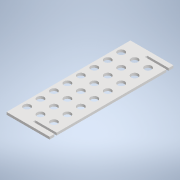
# Autodesk Inventor part: ChromoHolder
Saved by Autodesk Inventor 2020 (Build 240168000, 168)
## iProperties
Created: 2019-07-01
Part Number: ChromoHolder
Material: Generic
Document SubType Name: Modeling
Designer: eugen
Density: 1 g/cm^3
Appearance: Default
Author: eugen
Autodesk Inventor part; units mm, degrees
ref_plane "YZ Plane" through (0, 0, 0) normal (1, 0, 0) x (0, 1, 0)
ref_plane "XZ Plane" through (0, 0, 0) normal (0, 1, 0) x (-1, 0, 0)
ref_plane "XY Plane" through (0, 0, 0) normal (0, 0, 1) x (1, 0, 0)
sketch "Sketch1" plane through (0, 0, 0) normal (0, 1, 0) x (-1, 0, 0)
  line L0 (0, 0) -> (112.903, 0)
  line L1 (112.903, 0) -> (112.903, -324.7199)
  line L2 (112.903, -324.7199) -> (0, -324.7199)
  line L3 (0, -324.7199) -> (0, 0)
  line L4 (112.903, -0.6921) -> (112.903, 5.2769)
  line L5 (0, -12.7) -> (55.1815, -12.7)
  line L6 (56.4515, -13.97) -> (56.4515, -17.272)
  line L7 (55.1815, -18.542) -> (0, -18.542)
  line L8 (0, -18.542) -> (0, -12.7)
  line L9 (112.903, -312.0199) -> (112.903, -306.051)
  line L10 (0, -312.0199) -> (55.1815, -312.0199)
  line L11 (56.4515, -310.75) -> (56.4515, -307.4479)
  line L12 (55.1815, -306.1779) -> (0, -306.178)
  line L13 (0, -306.178) -> (0, -312.0199)
  circle A0 centre (62.8015, -38.9668) radius 9.1281
  line L14 (62.8015, 0) -> (62.8015, -324.7199) construction
  line L15 (27.5463, 0) -> (27.5463, -324.7199) construction
  circle A1 centre (62.8015, -74.222) radius 9.1281
  circle A2 centre (62.8015, -109.4772) radius 9.1281
  circle A3 centre (62.8015, -144.7324) radius 9.1281
  circle A4 centre (62.8015, -179.9876) radius 9.1281
  circle A5 centre (62.8015, -215.2428) radius 9.1281
  circle A6 centre (62.8015, -250.498) radius 9.1281
  circle A7 centre (62.8015, -285.7532) radius 9.1281
  circle A8 centre (27.5463, -38.9668) radius 9.1281
  circle A9 centre (27.5463, -74.222) radius 9.1281
  circle A10 centre (27.5463, -109.4772) radius 9.1281
  circle A11 centre (27.5463, -144.7324) radius 9.1281
  circle A12 centre (27.5463, -179.9876) radius 9.1281
  circle A13 centre (27.5463, -215.2428) radius 9.1281
  circle A14 centre (27.5463, -250.498) radius 9.1281
  circle A15 centre (27.5463, -285.7532) radius 9.1281
  line L16 (98.0567, -306.051) -> (98.0567, -0.6921) construction
  circle A16 centre (98.0567, -38.9668) radius 9.1281
  circle A17 centre (98.0567, -74.222) radius 9.1281
  circle A18 centre (98.0567, -109.4772) radius 9.1281
  circle A19 centre (98.0567, -144.7324) radius 9.1281
  circle A20 centre (98.0567, -179.9876) radius 9.1281
  circle A21 centre (98.0567, -215.2428) radius 9.1281
  circle A22 centre (98.0567, -250.498) radius 9.1281
  circle A23 centre (98.0567, -285.7532) radius 9.1281
  line L17 (27.5463, -38.9668) -> (98.0567, -38.9668) construction
  arc A24 (55.1815, -312.0199) -> (56.4515, -310.75) centre (55.1815, -310.75) ccw
  arc A25 (56.4515, -307.4479) -> (55.1815, -306.1779) centre (55.1815, -307.4479) ccw
  arc A26 (55.1815, -18.542) -> (56.4515, -17.272) centre (55.1815, -17.272) ccw
  arc A27 (56.4515, -13.97) -> (55.1815, -12.7) centre (55.1815, -13.97) ccw
  point P0 (56.4515, -18.542)
  point P1 (56.4515, -12.7)
  point P2 (56.4515, -306.178)
  point P3 (56.4515, -312.0199)
  point P4 (0, -18.542)
  point P5 (0, -306.178)
  point P6 (91.7067, -263.525)
  dimension "d10" = 35.2552
  dimension "d42" = 35.2552
  dimension "d0" = 112.903
  dimension "d1" = 324.7199
  dimension "d7" = 18.2563
  dimension "d11" = 35.2552
  dimension "d12" = 35.2552
  dimension "d13" = 35.2552
  dimension "d14" = 35.2552
  dimension "d15" = 35.2552
  dimension "d16" = 35.2552
  dimension "d17" = 35.2552
  dimension "d21" = 18.2563
  dimension "d22" = 35.2552
  dimension "d23" = 35.2552
  dimension "d24" = 35.2552
  dimension "d25" = 35.2552
  dimension "d26" = 35.2552
  dimension "d27" = 35.2552
  dimension "d28" = 35.2552
  dimension "d34" = 18.2563
  dimension "d35" = 35.2552
  dimension "d36" = 35.2552
  dimension "d37" = 35.2552
  dimension "d38" = 35.2552
  dimension "d39" = 35.2552
  dimension "d40" = 35.2552
  dimension "d41" = 35.2552
  dimension "d43" = 14.8463
  dimension "d48" = 5.842
  dimension "d49" = 5.842
  dimension "d50" = 56.4515
  dimension "d51" = 12.7
  dimension "d52" = 12.7
  dimension "d53" = 144.7324
  dimension "d54" = 1.27
  constraints: 30 end point, 28 centre point, 24 equal radius, 16 point on line, 8 point on circle, 8 tangent, 6 horizontal, 6 parallel, 3 perpendicular, 1 collinear, 1 midpoint, 32 other
  measures "d0" distance of L1.end L2.end
  measures "d1" distance of L0.end L1.end
  measures "d7" diameter of A0
  measures "d11" distance of A1.centre A0.centre
  measures "d12" distance of A2.centre A1.centre
  measures "d13" distance of A3.centre A2.centre
  measures "d14" distance of A4.centre A3.centre
  measures "d15" distance of A4.centre A5.centre
  measures "d16" distance of A6.centre A5.centre
  measures "d17" distance of A6.centre A7.centre
  measures "d21" diameter of A8
  measures "d22" distance of A9.centre L17.start
  measures "d23" distance of A10.centre A9.centre
  measures "d24" distance of A11.centre A10.centre
  measures "d25" distance of A12.centre A11.centre
  measures "d26" distance of A12.centre A13.centre
  measures "d27" distance of A14.centre A13.centre
  measures "d28" distance of A14.centre A15.centre
  measures "d34" diameter of A16
  measures "d35" distance of A17.centre L17.end
  measures "d36" distance of A18.centre A17.centre
  measures "d37" distance of A19.centre A18.centre
  measures "d38" distance of A20.centre A19.centre
  measures "d39" distance of A20.centre A21.centre
  measures "d40" distance of A22.centre A21.centre
  measures "d41" distance of A22.centre A23.centre
  measures "d48" distance between parallel lines of L10 L12
  measures "d49" distance between parallel lines of L7 L5
  measures "d50" distance between parallel lines of L3 L6
  measures "d51" distance between parallel lines of L0 L5
  measures "d52" distance between parallel lines of L2 L10
  measures "d53" distance from line of L0 A11.centre
  measures "d54" radius of A24
extrude "Extrusion1" add sketch "Sketch1" along normal blind 6.35 contours L0 L1 L2 L3 L10 A24 L11 A25 L12 L7 A26 L6 A27 L5
equation "\"d10\" = d11"
equation "\"d42\" = d35"
equation "\"d12\" = d11"
equation "\"d13\" = d11"
equation "\"d14\" = d11"
equation "\"d15\" = d11"
equation "\"d16\" = d11"
equation "\"d17\" = d11"
equation "\"d22\" = d11"
equation "\"d23\" = d22"
equation "\"d24\" = d22"
equation "\"d25\" = d22"
equation "\"d26\" = d22"
equation "\"d27\" = d22"
equation "\"d28\" = d22"
equation "\"d36\" = d35"
equation "\"d37\" = d35"
equation "\"d38\" = d35"
equation "\"d39\" = d35"
equation "\"d40\" = d35"
equation "\"d41\" = d35"
body "Solid1"
